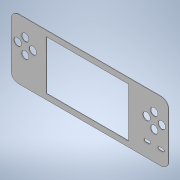
# Autodesk Inventor part: pannel
Saved by Autodesk Inventor 2022 (Build 260153000, 153)
## iProperties
Created: 2022-09-10
Part Number: pannel
Material: 常规
Document SubType Name: Modeling
Designer: ymc
Density: 1 g/cm^3
Appearance: 默认
Author: ymc
Autodesk Inventor part; units mm, degrees
ref_plane "YZ Plane" through (0, 0, 0) normal (1, 0, 0) x (0, 1, 0)
ref_plane "XZ Plane" through (0, 0, 0) normal (0, 1, 0) x (-1, 0, 0)
ref_plane "XY Plane" through (0, 0, 0) normal (0, 0, 1) x (1, 0, 0)
sketch "草图1" plane through (0, 0, 0) normal (0, 0, 1) x (1, 0, 0)
  line L0 (160.06, 15.83) -> (164.06, 15.83) construction
  line L1 (145.2, 15.83) -> (149.2, 15.83) construction
  line L2 (8.05, 0.05) -> (162, 0.05)
  line L3 (170, 8.05) -> (170, 57)
  line L4 (162, 65) -> (8.05, 65)
  line L5 (0.05, 57) -> (0.05, 8.05)
  line L6 (51, 0.05) -> (56.35, 0.05)
  line L7 (143.65, 15.83) -> (150.75, 15.83) construction
  line L8 (145.2, 14.28) -> (149.2, 14.28)
  line L9 (149.2, 17.38) -> (145.2, 17.38)
  arc A0 (145.2, 17.38) -> (145.2, 14.28) centre (145.2, 15.83) ccw
  arc A1 (149.2, 14.28) -> (149.2, 17.38) centre (149.2, 15.83) ccw
  line L10 (158.51, 15.83) -> (165.61, 15.83) construction
  line L11 (160.06, 14.28) -> (164.06, 14.28)
  line L12 (164.06, 17.38) -> (160.06, 17.38)
  arc A2 (160.06, 17.38) -> (160.06, 14.28) centre (160.06, 15.83) ccw
  arc A3 (164.06, 14.28) -> (164.06, 17.38) centre (164.06, 15.83) ccw
  arc A4 (8.05, 65) -> (0.05, 57) centre (8.05, 57) ccw
  arc A5 (0.05, 8.05) -> (8.05, 0.05) centre (8.05, 8.05) ccw
  arc A6 (162, 0.05) -> (170, 8.05) centre (162, 8.05) ccw
  arc A7 (170, 57) -> (162, 65) centre (162, 57) ccw
  line L13 (126.7, 5.88) -> (38.15, 5.88)
  line L14 (38.15, 5.88) -> (38.15, 59.12)
  line L15 (38.15, 59.12) -> (126.7, 59.12)
  line L16 (126.7, 59.12) -> (126.7, 5.88)
  circle A8 centre (154.65, 30.5) radius 4.05
  circle A9 centre (162.9, 38.75) radius 4.05
  circle A10 centre (154.65, 47) radius 4.05
  circle A11 centre (146.4, 38.75) radius 4.05
  circle A12 centre (15.38, 47) radius 4.05
  circle A13 centre (7.13, 38.85) radius 4.05
  circle A14 centre (23.63, 38.85) radius 4.05
  circle A15 centre (15.38, 30.6) radius 4.05
  line L17 (13.9543, 51.1457) -> (13.9543, 54.4563) construction
  line L18 (13.9543, 54.4563) -> (16.2984, 54.4563) construction
  line L19 (16.2984, 54.4563) -> (16.2984, 51.1457) construction
  line L20 (16.2984, 51.1457) -> (13.9543, 51.1457) construction
  line L21 (27.9171, 39.8995) -> (30.9676, 39.8995) construction
  line L22 (30.9676, 39.8995) -> (30.9676, 37.5554) construction
  line L23 (30.9676, 37.5554) -> (27.9171, 37.5554) construction
  line L24 (27.9171, 37.5554) -> (27.9171, 39.8995) construction
  line L25 (17.0897, 26.4529) -> (17.0897, 23.4024) construction
  line L26 (17.0897, 23.4024) -> (14.7456, 23.4024) construction
  line L27 (14.7456, 23.4024) -> (14.7456, 26.4529) construction
  line L28 (14.7456, 26.4529) -> (17.0897, 26.4529) construction
  line L29 (3.2389, 37.4761) -> (0.1885, 37.4761) construction
  line L30 (0.1885, 37.4761) -> (0.1885, 39.8201) construction
  line L31 (0.1885, 39.8201) -> (3.2389, 39.8201) construction
  line L32 (3.2389, 39.8201) -> (3.2389, 37.4761) construction
  line L33 (160.4662, 33.5387) -> (163.0202, 33.5387) construction
  line L34 (163.0202, 33.5387) -> (163.0202, 30.4907) construction
  line L35 (163.0202, 30.4907) -> (160.4662, 30.4907) construction
  line L36 (160.4662, 30.4907) -> (160.4662, 33.5387) construction
  line L37 (150.6642, 24.81) -> (154.3505, 24.81) construction
  line L38 (154.3505, 24.81) -> (154.3505, 21.762) construction
  line L39 (154.3505, 21.762) -> (150.6642, 21.762) construction
  line L40 (150.6642, 21.762) -> (150.6642, 24.81) construction
  line L41 (139.4313, 35.6136) -> (142.3206, 35.6136) construction
  line L42 (142.3206, 35.6136) -> (142.3206, 32.5636) construction
  line L43 (142.3206, 32.5636) -> (139.4313, 32.5636) construction
  line L44 (139.4313, 32.5636) -> (139.4313, 35.6136) construction
  line L45 (146.4429, 47.8482) -> (148.8759, 47.8482) construction
  line L46 (148.8759, 47.8482) -> (148.8759, 44.8002) construction
  line L47 (148.8759, 44.8002) -> (146.4429, 44.8002) construction
  line L48 (146.4429, 44.8002) -> (146.4429, 47.8482) construction
  line L49 (143.1052, 12.826) -> (157.1942, 12.826) construction
  line L50 (157.1942, 12.826) -> (157.1942, 9.6693) construction
  line L51 (157.1942, 9.6693) -> (143.1052, 9.6693) construction
  line L52 (143.1052, 9.6693) -> (143.1052, 12.826) construction
  line L53 (158.2616, 12.7189) -> (170.6092, 12.7189) construction
  line L54 (170.6092, 12.7189) -> (170.6092, 9.5622) construction
  line L55 (170.6092, 9.5622) -> (158.2616, 9.5622) construction
  line L56 (158.2616, 9.5622) -> (158.2616, 12.7189) construction
  point P0 (0, 0)
  point P1 (0, 0)
  point P2 (162.06, 15.83)
  point P3 (147.2, 15.83)
  point P4 (72.9763, 65)
  point P5 (0, 0)
  point P6 (170, 65)
  point P7 (170, 0.05)
  point P8 (0.05, 65)
  point P9 (147.2, 15.83)
  point P10 (162.06, 15.83)
  dimension "d12" = 2
  dimension "d13" = 2
  dimension "d23" = 169.95
  dimension "d24" = 64.95
  dimension "d25" = 7.1
  dimension "d26" = 3.1
  dimension "d27" = 7.1
  dimension "d28" = 3.1
  dimension "d29" = 8
  dimension "d30" = 88.55
  dimension "d34" = 53.24
  dimension "d35" = 8.1
  dimension "d36" = 8.1
  dimension "d37" = 8.1
  dimension "d38" = 8.1
  dimension "d39" = 8.1
  dimension "d40" = 8.1
  dimension "d41" = 8.1
  dimension "d42" = 8.1
  constraints: 42 end point, 20 point on circle, 16 centre point, 16 tangent, 14 point on line, 5 horizontal, 4 midpoint, 4 parallel, 4 perpendicular, 3 equal radius, 30 other
  measures "d12" distance of point (162.06, 15.83) L0.end
  measures "d13" distance of point (147.2, 15.83) L1.end
  measures "d23" distance of point (0.05, 65) point (170, 65)
  measures "d24" distance of point (170, 65) point (170, 0.05)
  measures "d25" distance of L7.start L7.end
  measures "d26" diameter of A1
  measures "d27" distance of L10.start L10.end
  measures "d28" diameter of A3
  measures "d29" radius of A4
  measures "d30" distance of L13.start L13.end
  measures "d34" distance of L15.end L13.start
  measures "d35" diameter of A8
  measures "d36" diameter of A9
  measures "d37" diameter of A10
  measures "d38" diameter of A11
  measures "d39" diameter of A12
  measures "d40" diameter of A13
  measures "d41" diameter of A14
  measures "d42" diameter of A15
extrude "拉伸1" add sketch "草图1" along normal blind 0.5
